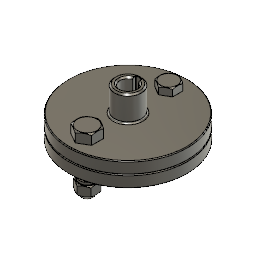
FlangeAssemblyGOST (Autodesk Fusion 360 design; units mm, degrees)
Autodesk Fusion 360 part; units mm, degrees
sketch "Sketch1" plane through (0, 0, 0) normal (0, 0, 1) x (1, 0, 0) in component "Полумуфта v5"
  line L0 (0, 0) -> (0, 1000)
  line L1 (0, 25) -> (9, 25)
  line L2 (9, 25) -> (9, 9)
  line L3 (10, 8) -> (40, 8)
  line L4 (40, 8) -> (40, 0)
  line L5 (40, 0) -> (0, 0)
  line L6 (0, 2) -> (12.5, 2)
  line L7 (12.5, 2) -> (12.5, 0)
  arc A0 (9, 9) -> (10, 8) centre (10, 9) ccw
  dimension "d3" = 80
  dimension "d4" = 25
  dimension "d10" = 18
  dimension "d12" = 2
  dimension "d13" = 8
  dimension "d14" = 25
  dimension "d39" = 1
  dimension "d70" = 1000
  constraint coincident L0.start L5.end
  constraint vertical L0
  constraint coincident L0 L1.start
  constraint perpendicular L0 L1
  constraint perpendicular L2 L3
  constraint perpendicular L3 L4
  constraint vertical L2
  constraint horizontal L5
  constraint coincident L0 L6.start
  constraint perpendicular L0 L6
  constraint coincident L5 L7.end
  constraint perpendicular L5 L7
  constraint tangent L2 A0
  constraint tangent L3 A0
  measures "d4" distance of L1 L5
  measures "d12" distance of L6.end L7.end
  measures "d13" distance of L3.end L4.end
  measures "d39" radius of A0
  measures "d70" distance of L0.start L0.end
revolve "Revolve1" add sketch "Sketch1" angle 360 about axis through (0, 0, 0) along (0, 1, 0) contours L0 L1 L2 L3 L4 L5 L6 L7 A0 makes body 1 in component "Полумуфта v5"
sketch "Sketch2" plane through (0, 25, 0) normal (0, 1, 0) x (-1, 0, 0) in component "Полумуфта v5"
  circle A0 centre (0, 0) radius 9
  circle A1 centre (0, 0) radius 5.5
  line L0 (0, 0) -> (0, -40.0415) construction
  line L1 (2, -5.1235) -> (2, -7.1)
  line L2 (1.8, -7.3) -> (0, -7.3)
  line L3 (0, 0) -> (0, 5.5) construction
  line L4 (0, -7.3) -> (-1.8, -7.3)
  line L5 (-2, -7.1) -> (-2, -5.1235)
  arc A2 (1.8, -7.3) -> (2, -7.1) centre (1.8, -7.1) ccw
  arc A3 (-2, -7.1) -> (-1.8, -7.3) centre (-1.8, -7.1) ccw
  point P0 (2, -7.3)
  dimension "d17" = 11
  dimension "d21" = 2
  dimension "d24" = 12.8
  dimension "d44" = 0.2
  constraint coincident A0.centre A1.centre
  constraint vertical L0
  constraint coincident A1 L1.start
  constraint vertical L1
  constraint coincident L0 L2.end
  constraint horizontal L2
  constraint coincident A1 L3.end
  constraint parallel L0 L3
  constraint perpendicular L0 L4
  constraint coincident A1 L5.end
  constraint perpendicular L4 L5
  constraint coincident P0 L2
  constraint coincident P0 L1
  constraint tangent L2 A2
  constraint tangent L1 A2
  constraint tangent L4 A3
  constraint tangent L5 A3
  constraint equal L1 L5
  constraint equal A2 A3
  measures "d17" diameter of A1
  measures "d21" distance of P0 L2.end
  measures "d24" distance of L2.end L3.end
  measures "d44" radius of A2
extrude "Extrude1" cut sketch "Sketch2" along normal mid plane 2000 contours A1 | A1 L1 L2 L4 L5 A2 A3 bodies 1 in component "Полумуфта v5"
sketch "Sketch3" plane through (0, 8, 0) normal (0, 1, 0) x (-1, 0, 0) in component "Полумуфта v5"
  circle A0 centre (0, 0) radius 40
  circle A1 centre (0, 0) radius 27.5 construction
  line L0 (0, -40) -> (0, 40) construction
  circle A2 centre (0, -27.5) radius 4
  circle A3 centre (0, 27.5) radius 4.5
  circle A4 centre (0, 0) radius 10
  dimension "d30" = 55
  dimension "d31" = 8
  dimension "d32" = 9
  constraint coincident A0.centre A1.centre
  constraint coincident A0 L0.start
  constraint coincident A0 L0.end
  constraint vertical L0
  constraint coincident A0.centre L0
  constraint coincident A1 A2.centre
  constraint coincident L0 A2.centre
  constraint coincident L0 A3.centre
  constraint coincident A1 A3.centre
  measures "d30" diameter of A1
  measures "d31" diameter of A2
  measures "d32" diameter of A3
extrude "Extrude2" cut sketch "Sketch3" along normal mid plane 2000 contours A2 | A3 bodies 1 in component "Полумуфта v5"
chamfer "Chamfer7" distance 1 angle 45 2 edges at (0, 25, 5.5) (-8.3909, 25, -3.2545) on bodies 1 in component "Полумуфта v5"
chamfer "Chamfer8" distance 0.5 angle 45 4 edges at (4.1955, 8, 29.1273) (3.7293, 8, -26.0535) (-37.2931, 8, -14.4646) (-37.2931, 0, -14.4646) on bodies 1 in component "Полумуфта v5"
sketch "Sketch1 (2)" plane through (0, 0, 0) normal (0, 0, 1) x (1, 0, 0) in component "Полумуфта v5 (1)"
  line L0 (0, 0) -> (0, 1000)
  line L1 (0, 25) -> (9, 25)
  line L2 (9, 25) -> (9, 9)
  line L3 (10, 8) -> (40, 8)
  line L4 (40, 8) -> (40, 0)
  line L5 (40, 0) -> (0, 0)
  line L6 (0, 2) -> (12.5, 2)
  line L7 (12.5, 2) -> (12.5, 0)
  arc A0 (9, 9) -> (10, 8) centre (10, 9) ccw
  dimension "d3_1" = 80
  dimension "d4_1" = 25
  dimension "d10_1" = 18
  dimension "d12_1" = 2
  dimension "d13_1" = 8
  dimension "d14_1" = 25
  dimension "d39_1" = 1
  dimension "d71" = 1000
  constraint coincident L0.start L5.end
  constraint vertical L0
  constraint coincident L0 L1.start
  constraint perpendicular L0 L1
  constraint perpendicular L2 L3
  constraint perpendicular L3 L4
  constraint vertical L2
  constraint horizontal L5
  constraint coincident L0 L6.start
  constraint perpendicular L0 L6
  constraint coincident L5 L7.end
  constraint perpendicular L5 L7
  constraint tangent L2 A0
  constraint tangent L3 A0
  measures "d4_1" distance of L1 L5
  measures "d12_1" distance of L6.end L7.end
  measures "d13_1" distance of L3.end L4.end
  measures "d39_1" radius of A0
  measures "d71" distance of L0.start L0.end
revolve "Revolve1'" add sketch "Sketch1 (2)" angle 360 about axis through (0, 0, 0) along (0, 1, 0) separate body contours L0 L1 L2 L3 L4 L5 L6 L7 A0 makes body 2 in component "Полумуфта v5 (1)"
sketch "Sketch2 (2)" plane through (0, 25, 0) normal (0, 1, 0) x (-1, 0, 0) in component "Полумуфта v5 (1)"
  circle A0 centre (0, 0) radius 9
  circle A1 centre (0, 0) radius 5.5
  line L0 (0, 0) -> (0, -40.0415) construction
  line L1 (2, -5.1235) -> (2, -7.1)
  line L2 (1.8, -7.3) -> (0, -7.3)
  line L3 (0, 0) -> (0, 5.5) construction
  line L4 (0, -7.3) -> (-1.8, -7.3)
  line L5 (-2, -7.1) -> (-2, -5.1235)
  arc A2 (1.8, -7.3) -> (2, -7.1) centre (1.8, -7.1) ccw
  arc A3 (-2, -7.1) -> (-1.8, -7.3) centre (-1.8, -7.1) ccw
  point P0 (2, -7.3)
  dimension "d17_1" = 11
  dimension "d21_1" = 2
  dimension "d24_1" = 12.8
  dimension "d44_1" = 0.2
  constraint coincident A0.centre A1.centre
  constraint vertical L0
  constraint coincident A1 L1.start
  constraint vertical L1
  constraint coincident L0 L2.end
  constraint horizontal L2
  constraint coincident A1 L3.end
  constraint parallel L0 L3
  constraint perpendicular L0 L4
  constraint coincident A1 L5.end
  constraint perpendicular L4 L5
  constraint coincident P0 L2
  constraint coincident P0 L1
  constraint tangent L2 A2
  constraint tangent L1 A2
  constraint tangent L4 A3
  constraint tangent L5 A3
  constraint equal L1 L5
  constraint equal A2 A3
  measures "d17_1" diameter of A1
  measures "d21_1" distance of P0 L2.end
  measures "d24_1" distance of L2.end L3.end
  measures "d44_1" radius of A2
extrude "Extrude1'" cut sketch "Sketch2 (2)" along normal mid plane 2000 contours A1 | A1 L1 L2 L4 L5 A2 A3 bodies 2 in component "Полумуфта v5 (1)"
sketch "Sketch3 (2)" plane through (0, 8, 0) normal (0, 1, 0) x (-1, 0, 0) in component "Полумуфта v5 (1)"
  circle A0 centre (0, 0) radius 40
  circle A1 centre (0, 0) radius 27.5 construction
  line L0 (0, -40) -> (0, 40) construction
  circle A2 centre (0, -27.5) radius 4
  circle A3 centre (0, 27.5) radius 4.5
  circle A4 centre (0, 0) radius 10
  dimension "d30_1" = 55
  dimension "d31_1" = 8
  dimension "d32_1" = 9
  constraint coincident A0.centre A1.centre
  constraint coincident A0 L0.start
  constraint coincident A0 L0.end
  constraint vertical L0
  constraint coincident A0.centre L0
  constraint coincident A1 A2.centre
  constraint coincident L0 A2.centre
  constraint coincident L0 A3.centre
  constraint coincident A1 A3.centre
  measures "d30_1" diameter of A1
  measures "d31_1" diameter of A2
  measures "d32_1" diameter of A3
extrude "Extrude2'" cut sketch "Sketch3 (2)" along normal mid plane 2000 contours A2 | A3 bodies 2 in component "Полумуфта v5 (1)"
chamfer "Chamfer7'" distance 1 angle 45 2 edges at (0, 25, 5.5) (-8.3909, 25, -3.2545) on bodies 2 in component "Полумуфта v5 (1)"
chamfer "Chamfer8'" distance 0.5 angle 45 4 edges at (4.1955, 8, 29.1273) (3.7293, 8, -26.0535) (-37.2931, 8, -14.4646) (-37.2931, 0, -14.4646) on bodies 2 in component "Полумуфта v5 (1)"
sketch "Sketch1 (3)" plane through (0, 0, 0) normal (0, 1, 0) x (1, 0, 0) in component "БОЛТ ГОСТ 7796 v4"
  line L0 (0, 6.9282) -> (-6, 3.4641)
  line L1 (-6, 3.4641) -> (-6, -3.4641)
  line L2 (-6, -3.4641) -> (0, -6.9282)
  line L3 (0, -6.9282) -> (6, -3.4641)
  line L4 (6, -3.4641) -> (6, 3.4641)
  line L5 (6, 3.4641) -> (0, 6.9282)
  dimension "d2" = 12
  constraint vertical L4
  measures "d2" distance of L1 L4
extrude "Extrude1''" add sketch "Sketch1 (3)" along normal blind 5 separate body makes body 3 in component "БОЛТ ГОСТ 7796 v4"
sketch "Sketch2 (3)" plane through (0, 0, 0) normal (1, 0, 0) x (0, 0, -1) in component "БОЛТ ГОСТ 7796 v4"
  line L0 (-5.718, 5) -> (-7.8414, 5)
  line L1 (-7.8414, 5) -> (-7.8414, 3.774)
  line L2 (-7.8414, 3.774) -> (-5.718, 5)
  line L3 (0, 0) -> (0, 6.8651) construction
  point P0 (-3.4641, 5)
  dimension "d10_2" = 5.718
  dimension "d11" = 30
  constraint horizontal L0
  constraint perpendicular L0 L1
  constraint coincident L3.start origin
  constraint vertical L3
  constraint coincident L0 P0
  measures "d10_2" distance of L0.start L3
  measures "d11" angle of L0 L2
revolve "Revolve1''" cut sketch "Sketch2 (3)" angle 360 about axis through (0, 0, 0) along (0, 1, 0) bodies 3 in component "БОЛТ ГОСТ 7796 v4"
sketch "Sketch3 (3)" plane through (0, 0, 0) normal (1, 0, 0) x (0, 0, -1) in component "БОЛТ ГОСТ 7796 v4"
  line L0 (0, 6.1991) -> (0, -30)
  line L1 (-4, -0.2) -> (-4, -30)
  line L2 (-4, -30) -> (0, -30)
  line L3 (-4.2, 0) -> (-6.9208, 0) construction
  arc A0 (-4, -0.2) -> (-4.2, 0) centre (-4.2, -0.2) ccw
  line L4 (0, 0) -> (-6.9208, 0) construction
  line L5 (0, 0) -> (-4.2, 0)
  dimension "d17_2" = 8
  dimension "d26" = 0.2
  dimension "d27" = 30
  constraint vertical L0
  constraint coincident L4.start L0
  constraint vertical L1
  constraint horizontal L2
  constraint perpendicular L0 L3
  constraint tangent L3 A0
  constraint tangent L1 A0
  constraint coincident L4.start L5.start
  constraint perpendicular L0 L4
  measures "d26" radius of A0
  measures "d27" distance of L4.start L2
revolve "Revolve3" add sketch "Sketch3 (3)" angle 360 about axis through (0, 6.1991, 0) along (0, -1, 0) bodies 3 in component "БОЛТ ГОСТ 7796 v4"
thread "Thread3" "ISO Metric profile 9.0 M9x1 6g" major diameter 8 minor diameter 7 pitch 1 angle 60 resizes the face on face at (0.1994, -10.1333, 3.995) from (0, -30, 0) to (0, -8, 0) on bodies 3 in component "БОЛТ ГОСТ 7796 v4"
chamfer "Chamfer2" distance 0.5 angle 45 1 edges at (-3.7293, -30, 1.4465) on bodies 3 in component "БОЛТ ГОСТ 7796 v4"
sketch "Sketch1 (4)" plane through (0, 0, 0) normal (0, 1, 0) x (1, 0, 0) in component "Болт ГОСТ 7817 v6"
  line L0 (-7, 4.0415) -> (-7, -4.0415)
  line L1 (-7, -4.0415) -> (0, -8.0829)
  line L2 (0, -8.0829) -> (7, -4.0415)
  line L3 (7, -4.0415) -> (7, 4.0415)
  line L4 (7, 4.0415) -> (0, 8.0829)
  line L5 (0, 8.0829) -> (-7, 4.0415)
  dimension "d2_1" = 14
  constraint vertical L3
  measures "d2_1" distance of L0 L3
extrude "Extrude1'''" add sketch "Sketch1 (4)" along normal blind 6.5 separate body makes body 4 in component "Болт ГОСТ 7817 v6"
sketch "Sketch2 (4)" plane through (0, 0, 0) normal (1, 0, 0) x (0, 0, -1) in component "Болт ГОСТ 7817 v6"
  line L0 (6.671, 6.5) -> (9.8393, 6.5)
  line L1 (9.8393, 6.5) -> (9.8393, 4.6708)
  line L2 (9.8393, 4.6708) -> (6.671, 6.5)
  line L3 (0, 0) -> (0, 7.7268) construction
  point P0 (8.0829, 6.5)
  dimension "d6_1" = 6.671
  dimension "d7_1" = 30
  constraint horizontal L0
  constraint vertical L1
  constraint coincident L3.start origin
  constraint vertical L3
  constraint coincident L0 P0
  measures "d6_1" distance of L0.start L3
  measures "d7_1" angle of L0 L2
revolve "Revolve1'''" cut sketch "Sketch2 (4)" angle 360 about axis through (0, 0, 0) along (0, 1, 0) bodies 4 in component "Болт ГОСТ 7817 v6"
sketch "Sketch3 (4)" plane through (0, 0, 0) normal (1, 0, 0) x (0, 0, -1) in component "Болт ГОСТ 7817 v6"
  line L0 (0, 0) -> (0, -49.5853)
  line L1 (-5, -0.2) -> (-5, -21.634)
  line L2 (-5, -21.634) -> (-4.5, -22.5)
  line L3 (-4.5, -22.5) -> (-4.5, -34)
  line L4 (-4.5, -34) -> (-2.65, -34)
  line L5 (-2.65, -34) -> (-2.65, -35)
  line L6 (-2.65, -35) -> (0, -35)
  arc A0 (-5, -0.2) -> (-5.2, 0) centre (-5.2, -0.2) ccw
  line L7 (0, 0) -> (-5.2, 0)
  dimension "d17_3" = 35
  dimension "d19_2" = 10
  dimension "d20_2" = 9
  dimension "d21_2" = 1
  dimension "d22" = 30
  dimension "d25" = 5.3
  dimension "d26_1" = 0.2
  dimension "d34_2" = 22.5
  constraint coincident L0.start L7.start
  constraint vertical L0
  constraint parallel L0 L1
  constraint parallel L1 L3
  constraint perpendicular L3 L4
  constraint perpendicular L4 L5
  constraint coincident L0 L6.end
  constraint perpendicular L0 L6
  constraint tangent L1 A0
  constraint tangent A0 L7
  constraint horizontal L7
  measures "d17_3" distance of L0.start L6.end
  measures "d21_2" distance of L4.end L5.end
  measures "d22" angle of L1 L2
  measures "d26_1" radius of A0
  measures "d34_2" distance of L2.end L7
revolve "Revolve2" add sketch "Sketch3 (4)" angle 360 about axis through (0, 0, 0) along (0, -1, 0) bodies 4 in component "Болт ГОСТ 7817 v6"
sketch "Sketch4" plane through (0, 0, 0) normal (0, 0, 1) x (1, 0, 0) in component "Болт ГОСТ 7817 v6"
  line L0 (0, 0) -> (0, -35.5194) construction
  circle A0 centre (0, -29.5) radius 1
  dimension "d29_1" = 2
  dimension "d30_3" = 29.5
  constraint coincident L0.start origin
  constraint vertical L0
  constraint coincident L0 A0.centre
  measures "d29_1" diameter of A0
  measures "d30_3" distance of L0.start A0.centre
extrude "Extrude2''" cut sketch "Sketch4" along normal mid plane 200 bodies 4 in component "Болт ГОСТ 7817 v6"
thread "Thread1" "ISO Metric profile 8.0 M8x1.25 6g" major diameter 7.866 minor diameter 6.4455 pitch 1.25 angle 60 resizes the face on face at (-1.6435, -28.677, -4.1892) on bodies 4 in component "Болт ГОСТ 7817 v6"
sketch "Sketch1 (5)" plane through (0, 0, 0) normal (0, 1, 0) x (1, 0, 0) in component "Гайка ГОСТ 15521 v4"
  line L0 (-6, 3.4641) -> (-6, -3.4641)
  line L1 (-6, -3.4641) -> (0, -6.9282)
  line L2 (0, -6.9282) -> (6, -3.4641)
  line L3 (6, -3.4641) -> (6, 3.4641)
  line L4 (6, 3.4641) -> (0, 6.9282)
  line L5 (0, 6.9282) -> (-6, 3.4641)
  circle A0 centre (0, 0) radius 4
  dimension "d1" = 12
  dimension "d4_3" = 8
  constraint coincident A0.centre origin
  constraint vertical L3
  constraint vertical L0
  measures "d1" distance of L0 L3
  measures "d4_3" diameter of A0
extrude "Extrude1''''" add sketch "Sketch1 (5)" along normal blind 6.5 separate body makes body 5 in component "Гайка ГОСТ 15521 v4"
sketch "Sketch3 (5)" plane through (0, 0, 0) normal (1, 0, 0) x (0, 0, -1) in component "Гайка ГОСТ 15521 v4"
  line L0 (-5.718, 6.5) -> (-7.669, 6.5)
  line L1 (-7.669, 6.5) -> (-7.669, 5.3736)
  line L2 (-7.669, 5.3736) -> (-5.718, 6.5)
  line L3 (0, 0) -> (0, 8.4615)
  point P0 (0, 6.5)
  point P1 (-6.9282, 6.5)
  dimension "d9" = 5.718
  dimension "d10_3" = 30
  constraint horizontal L0
  constraint perpendicular L0 L1
  constraint coincident L3.start origin
  constraint perpendicular L0 L3
  constraint coincident L0 P1
  measures "d9" distance of L0.start L3
  measures "d10_3" angle of L0 L2
revolve "Revolve1''''" cut sketch "Sketch3 (5)" angle 360 about axis through (0, 0, 0) along (0, 1, 0) bodies 5 in component "Гайка ГОСТ 15521 v4"
ref_plane "WorkPlane1" through (0, 3.25, 0) normal (0, -1, 0) x (-1, 0, 0) in component "Гайка ГОСТ 15521 v4"
mirror "Mirror1" about plane through (0, 3.25, 0) normal (0, -1, 0) of 1 faces at (-5.3401, 6.1286, 3.4569) on bodies 5 in component "Гайка ГОСТ 15521 v4"
thread "Thread1'" "ISO Metric profile 8.0 M8x1.25 6H" major diameter 8 minor diameter 6 pitch 1 angle 60 resizes the face on face at (3.9801, 4.3333, 0.3983) on bodies 5 in component "Гайка ГОСТ 15521 v4"
chamfer "Chamfer1" distance 0.5 angle 45 2 edges at (-2.797, 6.5, -1.0848) (-2.797, 0, -1.0848) 1 faces at (2.9851, 4.3333, 0.2987) on bodies 5 in component "Гайка ГОСТ 15521 v4"
sketch "Sketch1 (6)" plane through (0, 0, 0) normal (0, 1, 0) x (1, 0, 0) in component "Гайка ГОСТ 15521 v4 (1)"
  line L0 (-6, 3.4641) -> (-6, -3.4641)
  line L1 (-6, -3.4641) -> (0, -6.9282)
  line L2 (0, -6.9282) -> (6, -3.4641)
  line L3 (6, -3.4641) -> (6, 3.4641)
  line L4 (6, 3.4641) -> (0, 6.9282)
  line L5 (0, 6.9282) -> (-6, 3.4641)
  circle A0 centre (0, 0) radius 4
  dimension "d1_1" = 12
  dimension "d4_4" = 8
  constraint coincident A0.centre origin
  constraint vertical L3
  constraint vertical L0
  measures "d1_1" distance of L0 L3
  measures "d4_4" diameter of A0
extrude "Extrude1'''''" add sketch "Sketch1 (6)" along normal blind 6.5 separate body makes body 6 in component "Гайка ГОСТ 15521 v4 (1)"
sketch "Sketch3 (6)" plane through (0, 0, 0) normal (1, 0, 0) x (0, 0, -1) in component "Гайка ГОСТ 15521 v4 (1)"
  line L0 (-5.718, 6.5) -> (-7.669, 6.5)
  line L1 (-7.669, 6.5) -> (-7.669, 5.3736)
  line L2 (-7.669, 5.3736) -> (-5.718, 6.5)
  line L3 (0, 0) -> (0, 8.4615)
  point P0 (0, 6.5)
  point P1 (-6.9282, 6.5)
  dimension "d9_1" = 5.718
  dimension "d10_4" = 30
  constraint horizontal L0
  constraint perpendicular L0 L1
  constraint coincident L3.start origin
  constraint perpendicular L0 L3
  constraint coincident L0 P1
  measures "d9_1" distance of L0.start L3
  measures "d10_4" angle of L0 L2
revolve "Revolve1'''''" cut sketch "Sketch3 (6)" angle 360 about axis through (0, 0, 0) along (0, 1, 0) bodies 6 in component "Гайка ГОСТ 15521 v4 (1)"
ref_plane "WorkPlane1" through (0, 3.25, 0) normal (0, -1, 0) x (-1, 0, 0) in component "Гайка ГОСТ 15521 v4 (1)"
mirror "Mirror1'" about plane through (0, 3.25, 0) normal (0, -1, 0) of 1 faces at (-5.3401, 6.1286, 3.4569) on bodies 6 in component "Гайка ГОСТ 15521 v4 (1)"
thread "Thread1''" "ISO Metric profile 8.0 M8x1.25 6H" major diameter 8 minor diameter 6 pitch 1 angle 60 resizes the face on face at (3.9801, 4.3333, 0.3983) on bodies 6 in component "Гайка ГОСТ 15521 v4 (1)"
chamfer "Chamfer1'" distance 0.5 angle 45 2 edges at (-2.797, 6.5, -1.0848) (-2.797, 0, -1.0848) 1 faces at (2.9851, 4.3333, 0.2987) on bodies 6 in component "Гайка ГОСТ 15521 v4 (1)"
sketch "Sketch1 (7)" plane through (0, 0, 0) normal (0, 1, 0) x (1, 0, 0) in component "Шайба ГОСТ 6402-78 v2"
  circle A0 centre (0, 0) radius 5.1
  circle A1 centre (0, 0) radius 4
  dimension "d7_4" = 10.2
  dimension "d8_1" = 8
  constraint coincident A0.centre A1.centre
  measures "d7_4" diameter of A0
  measures "d8_1" diameter of A1
extrude "Extrude1''''''" add sketch "Sketch1 (7)" along normal blind 1.6 separate body makes body 7 in component "Шайба ГОСТ 6402-78 v2"
sketch "Sketch2 (5)" plane through (0, 0, 0) normal (1, 0, 0) x (0, 0, -1) in component "Шайба ГОСТ 6402-78 v2"
  line L0 (0, 0) -> (0.5823, 1.6)
  line L1 (0.5823, 1.6) -> (-0.2177, 1.6)
  line L2 (-0.2177, 1.6) -> (-0.8, 0)
  line L3 (-0.8, 0) -> (0, 0)
  line L4 (0, 0) -> (-3.973, 0)
  line L5 (0, 0) -> (1.1775, 0) construction
  dimension "d12_5" = 1.6
  dimension "d13_4" = 0.8
  dimension "d14_4" = 70.002
  constraint coincident L0.start L3.end
  constraint horizontal L1
  constraint parallel L1 L3
  constraint parallel L1 L4
  constraint parallel L3 L5
  constraint parallel L0 L2
  measures "d12_5" vertical distance of L0.start L0.end
  measures "d13_4" distance of L0.end L1.end
  measures "d14_4" angle of L0 L5
extrude "Extrude2'''" cut sketch "Sketch2 (5)" along normal blind 1000 bodies 7 in component "Шайба ГОСТ 6402-78 v2"
sketch "Sketch1 (8)" plane through (0, 0, 0) normal (0, 1, 0) x (1, 0, 0) in component "Шайба ГОСТ 6402-78 v2 (1)"
  circle A0 centre (0, 0) radius 5.1
  circle A1 centre (0, 0) radius 4
  dimension "d7_5" = 10.2
  dimension "d8_2" = 8
  constraint coincident A0.centre A1.centre
  measures "d7_5" diameter of A0
  measures "d8_2" diameter of A1
extrude "Extrude1'''''''" add sketch "Sketch1 (8)" along normal blind 1.6 separate body makes body 8 in component "Шайба ГОСТ 6402-78 v2 (1)"
sketch "Sketch2 (6)" plane through (0, 0, 0) normal (1, 0, 0) x (0, 0, -1) in component "Шайба ГОСТ 6402-78 v2 (1)"
  line L0 (0, 0) -> (0.5823, 1.6)
  line L1 (0.5823, 1.6) -> (-0.2177, 1.6)
  line L2 (-0.2177, 1.6) -> (-0.8, 0)
  line L3 (-0.8, 0) -> (0, 0)
  line L4 (0, 0) -> (-3.973, 0)
  line L5 (0, 0) -> (1.1775, 0) construction
  dimension "d12_6" = 1.6
  dimension "d13_5" = 0.8
  dimension "d14_5" = 70.002
  constraint coincident L0.start L3.end
  constraint horizontal L1
  constraint parallel L1 L3
  constraint parallel L1 L4
  constraint parallel L3 L5
  constraint parallel L0 L2
  measures "d12_6" vertical distance of L0.start L0.end
  measures "d13_5" distance of L0.end L1.end
  measures "d14_5" angle of L0 L5
extrude "Extrude2''''" cut sketch "Sketch2 (6)" along normal blind 1000 bodies 8 in component "Шайба ГОСТ 6402-78 v2 (1)"
component "Полумуфта v5" placed x (1, 0, 0) y (0, 1, 0) z (0, 0, 1) at (0, 0, 0)
component "Полумуфта v5 (1)" placed x (-1, 0, 0) y (0, -1, 0) z (0, 0, 1) at (0, 0, 0)
component "БОЛТ ГОСТ 7796 v4" placed x (1, 0, 0) y (0, 1, 0) z (0, 0, 1) at (0, 8.2, -27.5)
component "Болт ГОСТ 7817 v6" placed x (1, 0, 0) y (0, 1, 0) z (0, 0, 1) at (0, 8.2, 27.5)
component "Гайка ГОСТ 15521 v4" placed x (1, 0, 0) y (0, 1, 0) z (0, 0, 1) at (0, -23.3821, 27.5)
component "Гайка ГОСТ 15521 v4 (1)" placed x (1, 0, 0) y (0, 1, 0) z (0, 0, 1) at (0, -16.1, -27.5)
component "Шайба ГОСТ 6402-78 v2" placed x (1, 0, 0) y (0, 1, 0) z (0, 0, 1) at (0, -16.8821, 27.5)
component "Шайба ГОСТ 6402-78 v2 (1)" placed x (1, 0, 0) y (0, 1, 0) z (0, 0, 1) at (0, -9.6, -27.5)
equation "DHC = 80 mm"
equation "LHC = 25 mm"
equation "d3 = DHC"
equation "d4 = LHC"
equation "l1HC = 8 mm"
equation "l2HC = 2 mm"
equation "d2HC = 25 mm"
equation "d1HC = 11 mm"
equation "d10 = dHC"
equation "d12 = l2HC"
equation "d13 = l1HC"
equation "d14 = d2HC"
equation "dHC = 18 mm"
equation "d17 = d1HC"
equation "ext_all_HC = 1000 mm"
equation "d19 = ext_all_HC"
equation "d21 = B_HC"
equation "B_HC = 2 mm"
equation "H_HC = 12.8 mm"
equation "d24 = H_HC"
equation "d3HC = 8 mm"
equation "d4HC = 9 mm"
equation "D2_HC = 55 mm"
equation "b1HC = 1 mm"
equation "b2HC = 0.5 mm"
equation "d30 = D2_HC"
equation "d31 = d3HC"
equation "d32 = d4HC"
equation "d33 = ext_all_HC"
equation "R1_HC = 1 mm"
equation "d39 = R1_HC"
equation "R_HC = 0.2 mm"
equation "d44 = R_HC"
equation "d49 = b1HC"
equation "d50 = b2HC"
equation "DHC2 = 80 mm"
equation "LHC2 = 25 mm"
equation "d3_1 = DHC2"
equation "d4_1 = LHC2"
equation "l1_HC2 = 8 mm"
equation "l2_HC2 = 2 mm"
equation "d2_HC2 = 25 mm"
equation "d1_HC2 = 11 mm"
equation "d10_1 = dHC2"
equation "d12_1 = l2_HC2"
equation "d13_1 = l1_HC2"
equation "d14_1 = d2_HC2"
equation "dHC2 = 18 mm"
equation "d17_1 = d1_HC2"
equation "ext_all_HC2 = 1000 mm"
equation "d19_1 = ext_all_HC2"
equation "d21_1 = B_HC2"
equation "B_HC2 = 2 mm"
equation "H_HC2 = 12.8 mm"
equation "d24_1 = H_HC2"
equation "d3HC2 = 8 mm"
equation "d4HC2 = 9 mm"
equation "D2_HC2 = 55 mm"
equation "b1_HC2 = 1 mm"
equation "b2_HC2 = 0.5 mm"
equation "d30_1 = D2_HC2"
equation "d31_1 = d3HC2"
equation "d32_1 = d4HC2"
equation "d33_1 = ext_all_HC2"
equation "R1_HC2 = 1 mm"
equation "d39_1 = R1_HC2"
equation "R_HC2 = 0.2 mm"
equation "d44_1 = R_HC2"
equation "d49_1 = b1_HC2"
equation "d50_1 = b2_HC2"
equation "S_bolt77 = 12 mm"
equation "d2 = S_bolt77"
equation "d_bolt77 = 8 mm"
equation "m_bolt77 = 5 mm"
equation "d6 = m_bolt77"
equation "D_bolt77 = 5.718 mm"
equation "d10_2 = D_bolt77"
equation "d11 = angle_30"
equation "l1_bolt77 = 30 mm"
equation "b_bolt77 = 22 mm"
equation "d17_2 = d_bolt77"
equation "chm_bolt77 = 0.5 mm"
equation "thr_bolt77 = 8 mm"
equation "d26 = R_bolt77"
equation "d27 = l1_bolt77"
equation "d30_2 = b_bolt77"
equation "d31_2 = chm_bolt77"
equation "S_bolt78 = 14 mm"
equation "d2_1 = S_bolt78"
equation "m_bolt78 = 6.5 mm"
equation "d4_2 = m_bolt78"
equation "d6_1 = ( S_bolt78 * 0.953 ) / 2"
equation "L_bolt78 = 35 mm"
equation "l1_bolt78 = 29.5 mm"
equation "l2_bolt78 = 22.5 mm"
equation "d_bolt78 = 9 mm"
equation "d1_bolt78 = 10 mm"
equation "R_bolt78 = 0.2 mm"
equation "l3_bolt78 = 1 mm"
equation "d17_3 = L_bolt78"
equation "d19_2 = d1_bolt78"
equation "d20_2 = d_bolt78"
equation "d21_2 = l3_bolt78"
equation "d3_bolt78 = 5.3 mm"
equation "d4_bolt78 = 2 mm"
equation "d25 = d3_bolt78"
equation "d26_1 = R_bolt78"
equation "ext_all_bolt = 100 mm"
equation "d29_1 = d4_bolt78"
equation "d30_3 = l1_bolt78"
equation "d31_3 = ext_all_bolt"
equation "d34_2 = l2_bolt78"
equation "bolt78_angle = 30 deg"
equation "d1 = S_nut"
equation "S_nut = 12 mm"
equation "d_nut = 8 mm"
equation "d4_3 = d_nut"
equation "k_nut = 6.5 mm"
equation "d6_2 = k_nut"
equation "d9 = ( 0.953 * S_nut ) / 2"
equation "d10_3 = angle_30"
equation "d13_2 = -k_nut / 2"
equation "ch_nut = 0.5 mm"
equation "d17_4 = ch_nut"
equation "nut_angle = 30 deg"
equation "d1_1 = S_nut2"
equation "S_nut2 = 12 mm"
equation "d_nut2 = 8 mm"
equation "d4_4 = d_nut2"
equation "k_nut2 = 6.5 mm"
equation "d6_3 = k_nut2"
equation "d9_1 = ( 0.953 * S_nut2 ) / 2"
equation "d10_4 = angle_30"
equation "d13_3 = -k_nut2 / 2"
equation "ch_nut2 = 0.5 mm"
equation "d17_5 = ch_nut2"
equation "nut_angle2 = 30 deg"
equation "d_ws = 8 mm"
equation "b_ws = 2 mm"
equation "Dws = 10.2 mm"
equation "Sws = 1.6 mm"
equation "angle_ws = 77.78 grad"
equation "ext_ws = 1000 mm"
equation "d7_4 = Dws"
equation "d8_1 = d_ws"
equation "d9_2 = Sws"
equation "d12_5 = Sws"
equation "d13_4 = Sws / 2"
equation "d14_4 = angle_ws"
equation "d15_4 = ext_ws"
equation "d_ws2 = 8 mm"
equation "b_ws2 = 2 mm"
equation "D_ws2 = 10.2 mm"
equation "Sws2 = 1.6 mm"
equation "angle_ws2 = 77.78 grad"
equation "ext_ws2 = 1000 mm"
equation "d7_5 = D_ws2"
equation "d8_2 = d_ws2"
equation "d9_3 = Sws2"
equation "d12_6 = Sws2"
equation "d13_5 = Sws2 / 2"
equation "d14_5 = angle_ws2"
equation "d15_5 = ext_ws2"
equation "R_bolt77 = 0.2 mm"
equation "DHC_1 = 80 mm"
equation "LHC_1 = 25 mm"
equation "l1HC_1 = 8 mm"
equation "l2HC_1 = 2 mm"
equation "d2HC_1 = 25 mm"
equation "d1HC_1 = 11 mm"
equation "dHC_1 = 18 mm"
equation "ext_all_HC_1 = 1000 mm"
equation "B_HC_1 = 2 mm"
equation "H_HC_1 = 12.8 mm"
equation "d3HC_1 = 8 mm"
equation "d4HC_1 = 9 mm"
equation "D2_HC_1 = 55 mm"
equation "b1HC_1 = 1 mm"
equation "b2HC_1 = 0.5 mm"
equation "R1_HC_1 = 1 mm"
equation "R_HC_1 = 0.2 mm"
equation "DHC2_1 = 80 mm"
equation "LHC2_1 = 25 mm"
equation "l1_HC2_1 = 8 mm"
equation "l2_HC2_1 = 2 mm"
equation "d2_HC2_1 = 25 mm"
equation "d1_HC2_1 = 11 mm"
equation "dHC2_1 = 18 mm"
equation "ext_all_HC2_1 = 1000 mm"
equation "B_HC2_1 = 2 mm"
equation "H_HC2_1 = 12.8 mm"
equation "d3HC2_1 = 8 mm"
equation "d4HC2_1 = 9 mm"
equation "D2_HC2_1 = 55 mm"
equation "b1_HC2_1 = 1 mm"
equation "b2_HC2_1 = 0.5 mm"
equation "R1_HC2_1 = 1 mm"
equation "R_HC2_1 = 0.2 mm"
equation "S_bolt77_1 = 12 mm"
equation "d_bolt77_1 = 8 mm"
equation "m_bolt77_1 = 5 mm"
equation "D_bolt77_1 = 5.718 mm"
equation "l1_bolt77_1 = 30 mm"
equation "b_bolt77_1 = 22 mm"
equation "chm_bolt77_1 = 0.5 mm"
equation "thr_bolt77_1 = 8 mm"
equation "S_bolt78_1 = 14 mm"
equation "m_bolt78_1 = 6.5 mm"
equation "L_bolt78_1 = 35 mm"
equation "l1_bolt78_1 = 29.5 mm"
equation "l2_bolt78_1 = 22.5 mm"
equation "d_bolt78_1 = 9 mm"
equation "d1_bolt78_1 = 10 mm"
equation "R_bolt78_1 = 0.2 mm"
equation "l3_bolt78_1 = 1 mm"
equation "d3_bolt78_1 = 5.3 mm"
equation "d4_bolt78_1 = 2 mm"
equation "ext_all_bolt_1 = 100 mm"
equation "bolt78_angle_1 = 30 deg"
equation "S_nut_1 = 12 mm"
equation "d_nut_1 = 8 mm"
equation "k_nut_1 = 6.5 mm"
equation "ch_nut_1 = 0.5 mm"
equation "nut_angle_1 = 30 deg"
equation "S_nut2_1 = 12 mm"
equation "d_nut2_1 = 8 mm"
equation "k_nut2_1 = 6.5 mm"
equation "ch_nut2_1 = 0.5 mm"
equation "nut_angle2_1 = 30 deg"
equation "d_ws_1 = 8 mm"
equation "b_ws_1 = 2 mm"
equation "Dws_1 = 10.2 mm"
equation "Sws_1 = 1.6 mm"
equation "angle_ws_1 = 77.78 grad"
equation "ext_ws_1 = 1000 mm"
equation "d_ws2_1 = 8 mm"
equation "b_ws2_1 = 2 mm"
equation "D_ws2_1 = 10.2 mm"
equation "Sws2_1 = 1.6 mm"
equation "angle_ws2_1 = 70 deg"
equation "ext_ws2_1 = 1000 mm"
equation "angle_30 = 30 deg"
equation "DHC_2 = 80 mm"
equation "LHC_2 = 25 mm"
equation "l1HC_2 = 8 mm"
equation "l2HC_2 = 2 mm"
equation "d2HC_2 = 25 mm"
equation "d1HC_2 = 11 mm"
equation "dHC_2 = 18 mm"
equation "ext_all_HC_2 = 1000 mm"
equation "B_HC_2 = 2 mm"
equation "H_HC_2 = 12.8 mm"
equation "d3HC_2 = 8 mm"
equation "d4HC_2 = 9 mm"
equation "D2_HC_2 = 55 mm"
equation "b1HC_2 = 1 mm"
equation "b2HC_2 = 0.5 mm"
equation "R1_HC_2 = 1 mm"
equation "R_HC_2 = 0.2 mm"
equation "DHC2_2 = 80 mm"
equation "LHC2_2 = 25 mm"
equation "l1_HC2_2 = 8 mm"
equation "l2_HC2_2 = 2 mm"
equation "d2_HC2_2 = 25 mm"
equation "d1_HC2_2 = 11 mm"
equation "dHC2_2 = 18 mm"
equation "ext_all_HC2_2 = 1000 mm"
equation "B_HC2_2 = 2 mm"
equation "H_HC2_2 = 12.8 mm"
equation "d3HC2_2 = 8 mm"
equation "d4HC2_2 = 9 mm"
equation "D2_HC2_2 = 55 mm"
equation "b1_HC2_2 = 1 mm"
equation "b2_HC2_2 = 0.5 mm"
equation "R1_HC2_2 = 1 mm"
equation "R_HC2_2 = 0.2 mm"
equation "S_bolt77_2 = 12 mm"
equation "d_bolt77_2 = 8 mm"
equation "m_bolt77_2 = 5 mm"
equation "D_bolt77_2 = 5.718 mm"
equation "l1_bolt77_2 = 30 mm"
equation "b_bolt77_2 = 22 mm"
equation "chm_bolt77_2 = 0.5 mm"
equation "thr_bolt77_2 = 8 mm"
equation "S_bolt78_2 = 14 mm"
equation "m_bolt78_2 = 6.5 mm"
equation "L_bolt78_2 = 35 mm"
equation "l1_bolt78_2 = 29.5 mm"
equation "l2_bolt78_2 = 22.5 mm"
equation "d_bolt78_2 = 9 mm"
equation "d1_bolt78_2 = 10 mm"
equation "R_bolt78_2 = 0.2 mm"
equation "l3_bolt78_2 = 1 mm"
equation "d3_bolt78_2 = 5.3 mm"
equation "d4_bolt78_2 = 2 mm"
equation "ext_all_bolt_2 = 100 mm"
equation "bolt78_angle_2 = 30 deg"
equation "S_nut_2 = 12 mm"
equation "d_nut_2 = 8 mm"
equation "k_nut_2 = 6.5 mm"
equation "ch_nut_2 = 0.5 mm"
equation "nut_angle_2 = 30 deg"
equation "S_nut2_2 = 12 mm"
equation "d_nut2_2 = 8 mm"
equation "k_nut2_2 = 6.5 mm"
equation "ch_nut2_2 = 0.5 mm"
equation "nut_angle2_2 = 30 deg"
equation "d_ws_2 = 8 mm"
equation "b_ws_2 = 2 mm"
equation "Dws_2 = 10.2 mm"
equation "Sws_2 = 1.6 mm"
equation "angle_ws_2 = 77.78 grad"
equation "ext_ws_2 = 1000 mm"
equation "d_ws2_2 = 8 mm"
equation "b_ws2_2 = 2 mm"
equation "D_ws2_2 = 10.2 mm"
equation "Sws2_2 = 1.6 mm"
equation "angle_ws2_2 = 77.78 grad"
equation "ext_ws2_2 = 1000 mm"
equation "R_bolt77_1 = 0.2 mm"
equation "DHC_1_1 = 80 mm"
equation "LHC_1_1 = 25 mm"
equation "l1HC_1_1 = 8 mm"
equation "l2HC_1_1 = 2 mm"
equation "d2HC_1_1 = 25 mm"
equation "d1HC_1_1 = 11 mm"
equation "dHC_1_1 = 18 mm"
equation "ext_all_HC_1_1 = 1000 mm"
equation "B_HC_1_1 = 2 mm"
equation "H_HC_1_1 = 12.8 mm"
equation "d3HC_1_1 = 8 mm"
equation "d4HC_1_1 = 9 mm"
equation "D2_HC_1_1 = 55 mm"
equation "b1HC_1_1 = 1 mm"
equation "b2HC_1_1 = 0.5 mm"
equation "R1_HC_1_1 = 1 mm"
equation "R_HC_1_1 = 0.2 mm"
equation "DHC2_1_1 = 80 mm"
equation "LHC2_1_1 = 25 mm"
equation "l1_HC2_1_1 = 8 mm"
equation "l2_HC2_1_1 = 2 mm"
equation "d2_HC2_1_1 = 25 mm"
equation "d1_HC2_1_1 = 11 mm"
equation "dHC2_1_1 = 18 mm"
equation "ext_all_HC2_1_1 = 1000 mm"
equation "B_HC2_1_1 = 2 mm"
equation "H_HC2_1_1 = 12.8 mm"
equation "d3HC2_1_1 = 8 mm"
equation "d4HC2_1_1 = 9 mm"
equation "D2_HC2_1_1 = 55 mm"
equation "b1_HC2_1_1 = 1 mm"
equation "b2_HC2_1_1 = 0.5 mm"
equation "R1_HC2_1_1 = 1 mm"
equation "R_HC2_1_1 = 0.2 mm"
equation "S_bolt77_1_1 = 12 mm"
equation "d_bolt77_1_1 = 8 mm"
equation "m_bolt77_1_1 = 5 mm"
equation "D_bolt77_1_1 = 5.718 mm"
equation "l1_bolt77_1_1 = 30 mm"
equation "b_bolt77_1_1 = 22 mm"
equation "chm_bolt77_1_1 = 0.5 mm"
equation "thr_bolt77_1_1 = 8 mm"
equation "S_bolt78_1_1 = 14 mm"
equation "m_bolt78_1_1 = 6.5 mm"
equation "L_bolt78_1_1 = 35 mm"
equation "l1_bolt78_1_1 = 29.5 mm"
equation "l2_bolt78_1_1 = 22.5 mm"
equation "d_bolt78_1_1 = 9 mm"
equation "d1_bolt78_1_1 = 10 mm"
equation "R_bolt78_1_1 = 0.2 mm"
equation "l3_bolt78_1_1 = 1 mm"
equation "d3_bolt78_1_1 = 5.3 mm"
equation "d4_bolt78_1_1 = 2 mm"
equation "ext_all_bolt_1_1 = 100 mm"
equation "bolt78_angle_1_1 = 30 deg"
equation "S_nut_1_1 = 12 mm"
equation "d_nut_1_1 = 8 mm"
equation "k_nut_1_1 = 6.5 mm"
equation "ch_nut_1_1 = 0.5 mm"
equation "nut_angle_1_1 = 30 deg"
equation "S_nut2_1_1 = 12 mm"
equation "d_nut2_1_1 = 8 mm"
equation "k_nut2_1_1 = 6.5 mm"
equation "ch_nut2_1_1 = 0.5 mm"
equation "nut_angle2_1_1 = 30 deg"
equation "d_ws_1_1 = 8 mm"
equation "b_ws_1_1 = 2 mm"
equation "Dws_1_1 = 10.2 mm"
equation "Sws_1_1 = 1.6 mm"
equation "angle_ws_1_1 = 77.78 grad"
equation "ext_ws_1_1 = 1000 mm"
equation "d_ws2_1_1 = 8 mm"
equation "b_ws2_1_1 = 2 mm"
equation "D_ws2_1_1 = 10.2 mm"
equation "Sws2_1_1 = 1.6 mm"
equation "angle_ws2_1_1 = 70 deg"
equation "ext_ws2_1_1 = 1000 mm"
equation "angle_30_1 = 30 deg"
equation "DHC_3 = 80 mm"
equation "LHC_3 = 25 mm"
equation "l1HC_3 = 8 mm"
equation "l2HC_3 = 2 mm"
equation "d2HC_3 = 25 mm"
equation "d1HC_3 = 11 mm"
equation "dHC_3 = 18 mm"
equation "ext_all_HC_3 = 1000 mm"
equation "B_HC_3 = 2 mm"
equation "H_HC_3 = 12.8 mm"
equation "d3HC_3 = 8 mm"
equation "d4HC_3 = 9 mm"
equation "D2_HC_3 = 55 mm"
equation "b1HC_3 = 1 mm"
equation "b2HC_3 = 0.5 mm"
equation "R1_HC_3 = 1 mm"
equation "R_HC_3 = 0.2 mm"
equation "DHC2_3 = 80 mm"
equation "LHC2_3 = 25 mm"
equation "l1_HC2_3 = 8 mm"
equation "l2_HC2_3 = 2 mm"
equation "d2_HC2_3 = 25 mm"
equation "d1_HC2_3 = 11 mm"
equation "dHC2_3 = 18 mm"
equation "ext_all_HC2_3 = 1000 mm"
equation "B_HC2_3 = 2 mm"
equation "H_HC2_3 = 12.8 mm"
equation "d3HC2_3 = 8 mm"
equation "d4HC2_3 = 9 mm"
equation "D2_HC2_3 = 55 mm"
equation "b1_HC2_3 = 1 mm"
equation "b2_HC2_3 = 0.5 mm"
equation "R1_HC2_3 = 1 mm"
equation "R_HC2_3 = 0.2 mm"
equation "S_bolt77_3 = 12 mm"
equation "d_bolt77_3 = 8 mm"
equation "m_bolt77_3 = 5 mm"
equation "D_bolt77_3 = 5.718 mm"
equation "l1_bolt77_3 = 30 mm"
equation "b_bolt77_3 = 22 mm"
equation "chm_bolt77_3 = 0.5 mm"
equation "thr_bolt77_3 = 8 mm"
equation "S_bolt78_3 = 14 mm"
equation "m_bolt78_3 = 6.5 mm"
equation "L_bolt78_3 = 35 mm"
equation "l1_bolt78_3 = 29.5 mm"
equation "l2_bolt78_3 = 22.5 mm"
equation "d_bolt78_3 = 9 mm"
equation "d1_bolt78_3 = 10 mm"
equation "R_bolt78_3 = 0.2 mm"
equation "l3_bolt78_3 = 1 mm"
equation "d3_bolt78_3 = 5.3 mm"
equation "d4_bolt78_3 = 2 mm"
equation "ext_all_bolt_3 = 100 mm"
equation "bolt78_angle_3 = 30 deg"
equation "S_nut_3 = 12 mm"
equation "d_nut_3 = 8 mm"
equation "k_nut_3 = 6.5 mm"
equation "ch_nut_3 = 0.5 mm"
equation "nut_angle_3 = 30 deg"
equation "S_nut2_3 = 12 mm"
equation "d_nut2_3 = 8 mm"
equation "k_nut2_3 = 6.5 mm"
equation "ch_nut2_3 = 0.5 mm"
equation "nut_angle2_3 = 30 deg"
equation "d_ws_3 = 8 mm"
equation "b_ws_3 = 2 mm"
equation "Dws_3 = 10.2 mm"
equation "Sws_3 = 1.6 mm"
equation "angle_ws_3 = 77.78 grad"
equation "ext_ws_3 = 1000 mm"
equation "d_ws2_3 = 8 mm"
equation "b_ws2_3 = 2 mm"
equation "D_ws2_3 = 10.2 mm"
equation "Sws2_3 = 1.6 mm"
equation "angle_ws2_3 = 77.78 grad"
equation "ext_ws2_3 = 1000 mm"
equation "R_bolt77_2 = 0.2 mm"
equation "DHC_1_2 = 80 mm"
equation "LHC_1_2 = 25 mm"
equation "l1HC_1_2 = 8 mm"
equation "l2HC_1_2 = 2 mm"
equation "d2HC_1_2 = 25 mm"
equation "d1HC_1_2 = 11 mm"
equation "dHC_1_2 = 18 mm"
equation "ext_all_HC_1_2 = 1000 mm"
equation "B_HC_1_2 = 2 mm"
equation "H_HC_1_2 = 12.8 mm"
equation "d3HC_1_2 = 8 mm"
equation "d4HC_1_2 = 9 mm"
equation "D2_HC_1_2 = 55 mm"
equation "b1HC_1_2 = 1 mm"
equation "b2HC_1_2 = 0.5 mm"
equation "R1_HC_1_2 = 1 mm"
equation "R_HC_1_2 = 0.2 mm"
equation "DHC2_1_2 = 80 mm"
equation "LHC2_1_2 = 25 mm"
equation "l1_HC2_1_2 = 8 mm"
equation "l2_HC2_1_2 = 2 mm"
equation "d2_HC2_1_2 = 25 mm"
equation "d1_HC2_1_2 = 11 mm"
equation "dHC2_1_2 = 18 mm"
equation "ext_all_HC2_1_2 = 1000 mm"
equation "B_HC2_1_2 = 2 mm"
equation "H_HC2_1_2 = 12.8 mm"
equation "d3HC2_1_2 = 8 mm"
equation "d4HC2_1_2 = 9 mm"
equation "D2_HC2_1_2 = 55 mm"
equation "b1_HC2_1_2 = 1 mm"
equation "b2_HC2_1_2 = 0.5 mm"
equation "R1_HC2_1_2 = 1 mm"
equation "R_HC2_1_2 = 0.2 mm"
equation "S_bolt77_1_2 = 12 mm"
equation "d_bolt77_1_2 = 8 mm"
equation "m_bolt77_1_2 = 5 mm"
equation "D_bolt77_1_2 = 5.718 mm"
equation "l1_bolt77_1_2 = 30 mm"
equation "b_bolt77_1_2 = 22 mm"
equation "chm_bolt77_1_2 = 0.5 mm"
equation "thr_bolt77_1_2 = 8 mm"
equation "S_bolt78_1_2 = 14 mm"
equation "m_bolt78_1_2 = 6.5 mm"
equation "L_bolt78_1_2 = 35 mm"
equation "l1_bolt78_1_2 = 29.5 mm"
equation "l2_bolt78_1_2 = 22.5 mm"
equation "d_bolt78_1_2 = 9 mm"
equation "d1_bolt78_1_2 = 10 mm"
equation "R_bolt78_1_2 = 0.2 mm"
equation "l3_bolt78_1_2 = 1 mm"
equation "d3_bolt78_1_2 = 5.3 mm"
equation "d4_bolt78_1_2 = 2 mm"
equation "ext_all_bolt_1_2 = 100 mm"
equation "bolt78_angle_1_2 = 30 deg"
equation "S_nut_1_2 = 12 mm"
equation "d_nut_1_2 = 8 mm"
equation "k_nut_1_2 = 6.5 mm"
equation "ch_nut_1_2 = 0.5 mm"
equation "nut_angle_1_2 = 30 deg"
equation "S_nut2_1_2 = 12 mm"
equation "d_nut2_1_2 = 8 mm"
equation "k_nut2_1_2 = 6.5 mm"
equation "ch_nut2_1_2 = 0.5 mm"
equation "nut_angle2_1_2 = 30 deg"
equation "d_ws_1_2 = 8 mm"
equation "b_ws_1_2 = 2 mm"
equation "Dws_1_2 = 10.2 mm"
equation "Sws_1_2 = 1.6 mm"
equation "angle_ws_1_2 = 77.78 grad"
equation "ext_ws_1_2 = 1000 mm"
equation "d_ws2_1_2 = 8 mm"
equation "b_ws2_1_2 = 2 mm"
equation "D_ws2_1_2 = 10.2 mm"
equation "Sws2_1_2 = 1.6 mm"
equation "angle_ws2_1_2 = 70 deg"
equation "ext_ws2_1_2 = 1000 mm"
equation "angle_30_2 = 30 deg"
equation "DHC_4 = 80 mm"
equation "LHC_4 = 25 mm"
equation "l1HC_4 = 8 mm"
equation "l2HC_4 = 2 mm"
equation "d2HC_4 = 25 mm"
equation "d1HC_4 = 11 mm"
equation "dHC_4 = 18 mm"
equation "ext_all_HC_4 = 1000 mm"
equation "B_HC_4 = 2 mm"
equation "H_HC_4 = 12.8 mm"
equation "d3HC_4 = 8 mm"
equation "d4HC_4 = 9 mm"
equation "D2_HC_4 = 55 mm"
equation "b1HC_4 = 1 mm"
equation "b2HC_4 = 0.5 mm"
equation "R1_HC_4 = 1 mm"
equation "R_HC_4 = 0.2 mm"
equation "DHC2_4 = 80 mm"
equation "LHC2_4 = 25 mm"
equation "l1_HC2_4 = 8 mm"
equation "l2_HC2_4 = 2 mm"
equation "d2_HC2_4 = 25 mm"
equation "d1_HC2_4 = 11 mm"
equation "dHC2_4 = 18 mm"
equation "ext_all_HC2_4 = 1000 mm"
equation "B_HC2_4 = 2 mm"
equation "H_HC2_4 = 12.8 mm"
equation "d3HC2_4 = 8 mm"
equation "d4HC2_4 = 9 mm"
equation "D2_HC2_4 = 55 mm"
equation "b1_HC2_4 = 1 mm"
equation "b2_HC2_4 = 0.5 mm"
equation "R1_HC2_4 = 1 mm"
equation "R_HC2_4 = 0.2 mm"
equation "S_bolt77_4 = 12 mm"
equation "d_bolt77_4 = 8 mm"
equation "m_bolt77_4 = 5 mm"
equation "D_bolt77_4 = 5.718 mm"
equation "l1_bolt77_4 = 30 mm"
equation "b_bolt77_4 = 22 mm"
equation "chm_bolt77_4 = 0.5 mm"
equation "thr_bolt77_4 = 8 mm"
equation "S_bolt78_4 = 14 mm"
equation "m_bolt78_4 = 6.5 mm"
equation "L_bolt78_4 = 35 mm"
equation "l1_bolt78_4 = 29.5 mm"
equation "l2_bolt78_4 = 22.5 mm"
equation "d_bolt78_4 = 9 mm"
equation "d1_bolt78_4 = 10 mm"
equation "R_bolt78_4 = 0.2 mm"
equation "l3_bolt78_4 = 1 mm"
equation "d3_bolt78_4 = 5.3 mm"
equation "d4_bolt78_4 = 2 mm"
equation "ext_all_bolt_4 = 100 mm"
equation "bolt78_angle_4 = 30 deg"
equation "S_nut_4 = 12 mm"
equation "d_nut_4 = 8 mm"
equation "k_nut_4 = 6.5 mm"
equation "ch_nut_4 = 0.5 mm"
equation "nut_angle_4 = 30 deg"
equation "S_nut2_4 = 12 mm"
equation "d_nut2_4 = 8 mm"
equation "k_nut2_4 = 6.5 mm"
equation "ch_nut2_4 = 0.5 mm"
equation "nut_angle2_4 = 30 deg"
equation "d_ws_4 = 8 mm"
equation "b_ws_4 = 2 mm"
equation "Dws_4 = 10.2 mm"
equation "Sws_4 = 1.6 mm"
equation "angle_ws_4 = 77.78 grad"
equation "ext_ws_4 = 1000 mm"
equation "d_ws2_4 = 8 mm"
equation "b_ws2_4 = 2 mm"
equation "D_ws2_4 = 10.2 mm"
equation "Sws2_4 = 1.6 mm"
equation "angle_ws2_4 = 77.78 grad"
equation "ext_ws2_4 = 1000 mm"
equation "R_bolt77_3 = 0.2 mm"
equation "DHC_1_3 = 80 mm"
equation "LHC_1_3 = 25 mm"
equation "l1HC_1_3 = 8 mm"
equation "l2HC_1_3 = 2 mm"
equation "d2HC_1_3 = 25 mm"
equation "d1HC_1_3 = 11 mm"
equation "dHC_1_3 = 18 mm"
equation "ext_all_HC_1_3 = 1000 mm"
equation "B_HC_1_3 = 2 mm"
equation "H_HC_1_3 = 12.8 mm"
equation "d3HC_1_3 = 8 mm"
equation "d4HC_1_3 = 9 mm"
equation "D2_HC_1_3 = 55 mm"
equation "b1HC_1_3 = 1 mm"
equation "b2HC_1_3 = 0.5 mm"
equation "R1_HC_1_3 = 1 mm"
equation "R_HC_1_3 = 0.2 mm"
equation "DHC2_1_3 = 80 mm"
equation "LHC2_1_3 = 25 mm"
equation "l1_HC2_1_3 = 8 mm"
equation "l2_HC2_1_3 = 2 mm"
equation "d2_HC2_1_3 = 25 mm"
equation "d1_HC2_1_3 = 11 mm"
equation "dHC2_1_3 = 18 mm"
equation "ext_all_HC2_1_3 = 1000 mm"
equation "B_HC2_1_3 = 2 mm"
equation "H_HC2_1_3 = 12.8 mm"
equation "d3HC2_1_3 = 8 mm"
equation "d4HC2_1_3 = 9 mm"
equation "D2_HC2_1_3 = 55 mm"
equation "b1_HC2_1_3 = 1 mm"
equation "b2_HC2_1_3 = 0.5 mm"
equation "R1_HC2_1_3 = 1 mm"
equation "R_HC2_1_3 = 0.2 mm"
equation "S_bolt77_1_3 = 12 mm"
equation "d_bolt77_1_3 = 8 mm"
equation "m_bolt77_1_3 = 5 mm"
equation "D_bolt77_1_3 = 5.718 mm"
equation "l1_bolt77_1_3 = 30 mm"
equation "b_bolt77_1_3 = 22 mm"
equation "chm_bolt77_1_3 = 0.5 mm"
equation "thr_bolt77_1_3 = 8 mm"
equation "S_bolt78_1_3 = 14 mm"
equation "m_bolt78_1_3 = 6.5 mm"
equation "L_bolt78_1_3 = 35 mm"
equation "l1_bolt78_1_3 = 29.5 mm"
equation "l2_bolt78_1_3 = 22.5 mm"
equation "d_bolt78_1_3 = 9 mm"
equation "d1_bolt78_1_3 = 10 mm"
equation "R_bolt78_1_3 = 0.2 mm"
equation "l3_bolt78_1_3 = 1 mm"
equation "d3_bolt78_1_3 = 5.3 mm"
equation "d4_bolt78_1_3 = 2 mm"
equation "ext_all_bolt_1_3 = 100 mm"
equation "bolt78_angle_1_3 = 30 deg"
equation "S_nut_1_3 = 12 mm"
equation "d_nut_1_3 = 8 mm"
equation "k_nut_1_3 = 6.5 mm"
equation "ch_nut_1_3 = 0.5 mm"
equation "nut_angle_1_3 = 30 deg"
equation "S_nut2_1_3 = 12 mm"
equation "d_nut2_1_3 = 8 mm"
equation "k_nut2_1_3 = 6.5 mm"
equation "ch_nut2_1_3 = 0.5 mm"
equation "nut_angle2_1_3 = 30 deg"
equation "d_ws_1_3 = 8 mm"
equation "b_ws_1_3 = 2 mm"
equation "Dws_1_3 = 10.2 mm"
equation "Sws_1_3 = 1.6 mm"
equation "angle_ws_1_3 = 77.78 grad"
equation "ext_ws_1_3 = 1000 mm"
equation "d_ws2_1_3 = 8 mm"
equation "b_ws2_1_3 = 2 mm"
equation "D_ws2_1_3 = 10.2 mm"
equation "Sws2_1_3 = 1.6 mm"
equation "angle_ws2_1_3 = 70 deg"
equation "ext_ws2_1_3 = 1000 mm"
equation "angle_30_3 = 30 deg"
